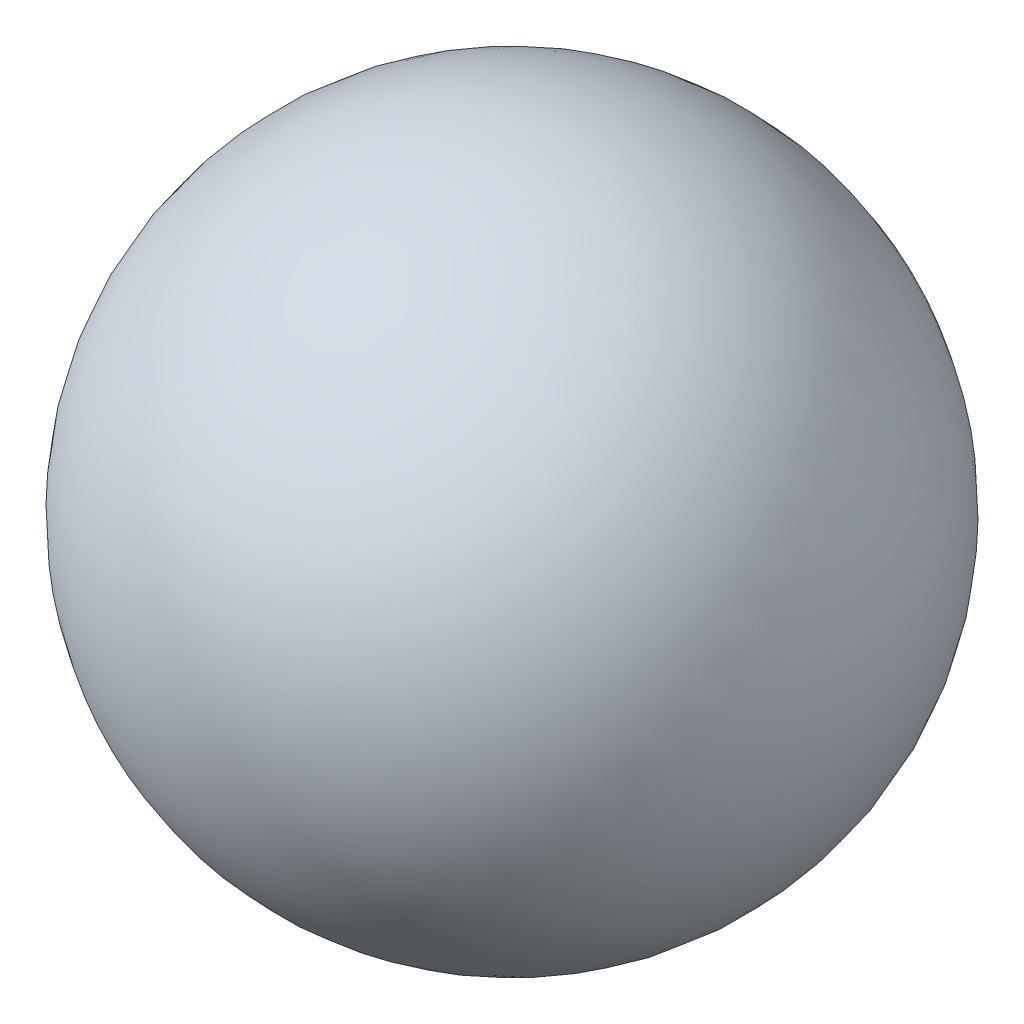
# Autodesk Inventor part: Glass Marble
Saved by Autodesk Inventor 2026.2 (Build 302298010, 298A)
## iProperties
Created: 2026-03-12
Part Number: Glass Marble
Material: Glass
Document SubType Name: Modeling
Designer: pjrah
Mass: 4.67536 g
Surface Area: 8.04248 cm^2
Volume: 2.14466 cm^3
Density: 2.18 g/cm^3
Appearance: Clear
Author: pjrah
Autodesk Inventor part; units mm, degrees
ref_plane "YZ Plane" through (0, 0, 0) normal (1, 0, 0) x (0, 1, 0)
ref_plane "XZ Plane" through (0, 0, 0) normal (0, 1, 0) x (-1, 0, 0)
ref_plane "XY Plane" through (0, 0, 0) normal (0, 0, 1) x (1, 0, 0)
sketch "Sketch1" plane through (0, 0, 0) normal (0, 0, 1) x (1, 0, 0)
  arc A0 (0, 8) -> (0, -8) centre (0, 0) ccw
  line L0 (0, 8) -> (0, -8)
  dimension "d0" = 16
  constraints: 2 end point, 2 point on circle, 1 centre point, 1 coincident, 1 vertical
  measures "d0" diameter of A0
revolve "Revolution1" add sketch "Sketch1" angle 360 about axis through (0, 8, 0) along (0, -1, 0)
body "Solid1"
